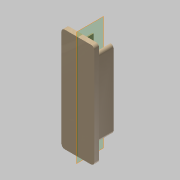
# Autodesk Inventor part: Maglock Aligner
Saved by Autodesk Inventor 2014 SP1 (Build 180222100, 222)
## iProperties
Created: 2014-01-09
Part Number: Maglock Aligner
Material: Polyethylene, High Density
Document SubType Name: Modeling
Designer: Rauhul Varma
Mass: 22.1615 g
Surface Area: 138.887 cm^2
Volume: 23.2789 cm^3
Density: 0.952 g/cm^3
Appearance: Smooth - Off-White
Author: Rauhul Varma
Autodesk Inventor part; units mm, degrees
ref_plane "YZ Plane" through (0, 0, 0) normal (1, 0, 0) x (0, 1, 0)
ref_plane "XZ Plane" through (0, 0, 0) normal (0, 1, 0) x (-1, 0, 0)
ref_plane "XY Plane" through (0, 0, 0) normal (0, 0, 1) x (1, 0, 0)
sketch "Sketch1" plane through (0, 0, 0) normal (0, 0, 1) x (1, 0, 0)
  line L0 (-18.6531, 0) -> (18.6531, 0)
  line L1 (18.6531, 0) -> (18.6531, 35.0141)
  line L2 (18.6531, 35.0141) -> (-18.6531, 35.0141)
  line L3 (-18.6531, 35.0141) -> (-18.6531, 0)
  line L4 (0, 0) -> (0, 35.0141) construction
  line L5 (-9.3266, 35.0141) -> (-9.3266, 0) construction
  line L6 (-1.8266, 0) -> (-1.8266, 145.5582) construction
  line L7 (-16.8266, 0) -> (-16.8266, 145.5582) construction
  line L8 (-16.8266, 145.5582) -> (-1.8266, 145.5582) construction
  line L9 (-25.4, 0) -> (25.4, 0) construction
  line L10 (25.4, 0) -> (25.4, 304.8) construction
  line L11 (25.4, 304.8) -> (-25.4, 304.8) construction
  line L12 (-25.4, 304.8) -> (-25.4, 0) construction
  line L13 (-25.4, 73.1141) -> (6.7469, 73.1141)
  line L14 (6.7469, 73.1141) -> (6.7469, 174.7141)
  line L15 (6.7469, 174.7141) -> (-25.4, 174.7141)
  line L16 (-25.4, 174.7141) -> (-25.4, 73.1141)
  line L17 (-20.6375, 85.8141) -> (1.9844, 85.8141)
  line L18 (1.9844, 85.8141) -> (1.9844, 162.0141)
  line L19 (1.9844, 162.0141) -> (-20.6375, 162.0141)
  line L20 (-20.6375, 162.0141) -> (-20.6375, 85.8141)
  line L21 (-17.4625, 162.0141) -> (-17.4625, 85.8141)
  line L22 (-1.1906, 85.8141) -> (-1.1906, 162.0141)
  line L23 (-15.6766, 168.3641) -> (-2.9766, 168.3641) construction
  line L24 (-15.6766, 171.5391) -> (-2.9766, 171.5391)
  line L25 (-2.9766, 165.1891) -> (-15.6766, 165.1891)
  arc A0 (-15.6766, 171.5391) -> (-15.6766, 165.1891) centre (-15.6766, 168.3641) ccw
  arc A1 (-2.9766, 165.1891) -> (-2.9766, 171.5391) centre (-2.9766, 168.3641) ccw
  line L26 (-15.6766, 79.4641) -> (-2.9766, 79.4641) construction
  line L27 (-15.6766, 76.2891) -> (-2.9766, 76.2891)
  line L28 (-2.9766, 82.6391) -> (-15.6766, 82.6391)
  arc A2 (-15.6766, 82.6391) -> (-15.6766, 76.2891) centre (-15.6766, 79.4641) ccw
  arc A3 (-2.9766, 76.2891) -> (-2.9766, 82.6391) centre (-2.9766, 79.4641) ccw
  point P0 (0, 0)
  point P1 (-9.3266, 168.3641)
  point P2 (-9.3266, 79.4641)
  dimension "d0" = 37.3062
  dimension "d1" = 35.0141
  dimension "d2" = 15
  dimension "d3" = 50.8
  dimension "d4" = 304.8
  dimension "d5" = 101.6
  dimension "d6" = 76.2
  dimension "d7" = 4.7625
  dimension "d8" = 4.7625
  dimension "d9" = 12.7
  dimension "d10" = 12.7
  dimension "d11" = 38.1
  dimension "d12" = 3.175
  dimension "d13" = 3.175
  dimension "d14" = 12.7
  dimension "d15" = 12.7
  dimension "d16" = 3.175
  dimension "d17" = 6.35
  dimension "d18" = 3.175
  dimension "d19" = 6.35
  constraints: 62 end point, 14 parallel, 11 point on line, 9 perpendicular, 8 point on circle, 8 tangent, 6 midpoint, 4 centre point, 4 horizontal, 5 other
  measures "d0" distance between parallel lines of L1 L3
  measures "d1" distance between parallel lines of L2 L0
  measures "d2" distance between parallel lines of L6 L7
  measures "d3" distance of L11.end L10.end
  measures "d4" distance of L10.end L9.end
  measures "d5" distance of L13.end L14.end
  measures "d6" distance between parallel lines of L17 L19
  measures "d7" distance between parallel lines of L12 L20
  measures "d8" distance between parallel lines of L14 L18
  measures "d9" distance between parallel lines of L15 L19
  measures "d10" distance between parallel lines of L13 L17
  measures "d11" distance between parallel lines of L2 L13
  measures "d12" distance between parallel lines of L20 L21
  measures "d13" distance between parallel lines of L18 L22
  measures "d14" distance of L26.start L26.end
  measures "d15" distance of L23.start L23.end
  measures "d16" radius of A2
  measures "d17" distance between parallel lines of L17 L26
  measures "d18" radius of A0
  measures "d19" distance between parallel lines of L19 L23
extrude "Extrusion1" add sketch "Sketch1" along normal blind 4.7625 contours L16 L15 L14 L13 | L20 L19 L21 L17 | L21 L19 L22 L17 | L22 L19 L18 L17 | L24 A1 L25 A0 | A2 L28 A3 L27
extrude "Extrusion2" cut sketch "Sketch1" along normal blind 2.3813 contours L24 A1 L25 A0 | A2 L28 A3 L27
extrude "Extrusion3" add sketch "Sketch1" against normal blind 19.05 contours L20 L19 L21 L17 | L22 L19 L18 L17
fillet "Fillet1" radius 3.175 8 edges at (-20.6375, 85.8141, -9.525) (1.9844, 85.8141, -9.525) (-20.6375, 162.0141, -9.525) (1.9844, 162.0141, -9.525) (6.7469, 73.1141, 2.3813) (-25.4, 73.1141, 2.3813) (-25.4, 174.7141, 2.3813) (6.7469, 174.7141, 2.3813)
ref_plane "Work Plane1" through (-9.3266, 85.8141, 0) normal (-1, 0, 0) x (0, 0, 1)
sketch "Sketch2" plane through (0, 0, -19.05) normal (0, 0, -1) x (-1, 0, 0)
  arc A0 (20.6375, 158.8391) -> (17.4625, 162.0141) centre (17.4625, 158.8391) ccw projected
  line L0 (17.4625, 162.0141) -> (17.4625, 85.8141) projected
  arc A1 (17.4625, 85.8141) -> (20.6375, 88.9891) centre (17.4625, 88.9891) ccw projected
  line L1 (20.6375, 88.9891) -> (20.6375, 158.8391) projected
  arc A2 (20.5105, 158.8391) -> (17.5895, 161.8844) centre (17.4625, 158.8391) ccw
  line L2 (20.5105, 158.8391) -> (20.5105, 88.9891)
  arc A3 (17.5895, 85.9437) -> (20.5105, 88.9891) centre (17.4625, 88.9891) ccw
  line L3 (17.5895, 85.9437) -> (17.5895, 161.8844)
  point P0 (0, 0)
  dimension "d27" = 0.127
  constraints: 4 end point, 4 point on circle, 2 centre point, 3 other
  measures "d27" distance between parallel lines of L1 L2
extrude "Extrusion4" cut sketch "Sketch2" against normal up to surface (19.05 mm away)
mirror "Mirror1" about plane through (-9.3266, 85.8141, 0) normal (-1, 0, 0) of "Extrusion4"
equation "\"d9\" = d10"
body "Solid1"
